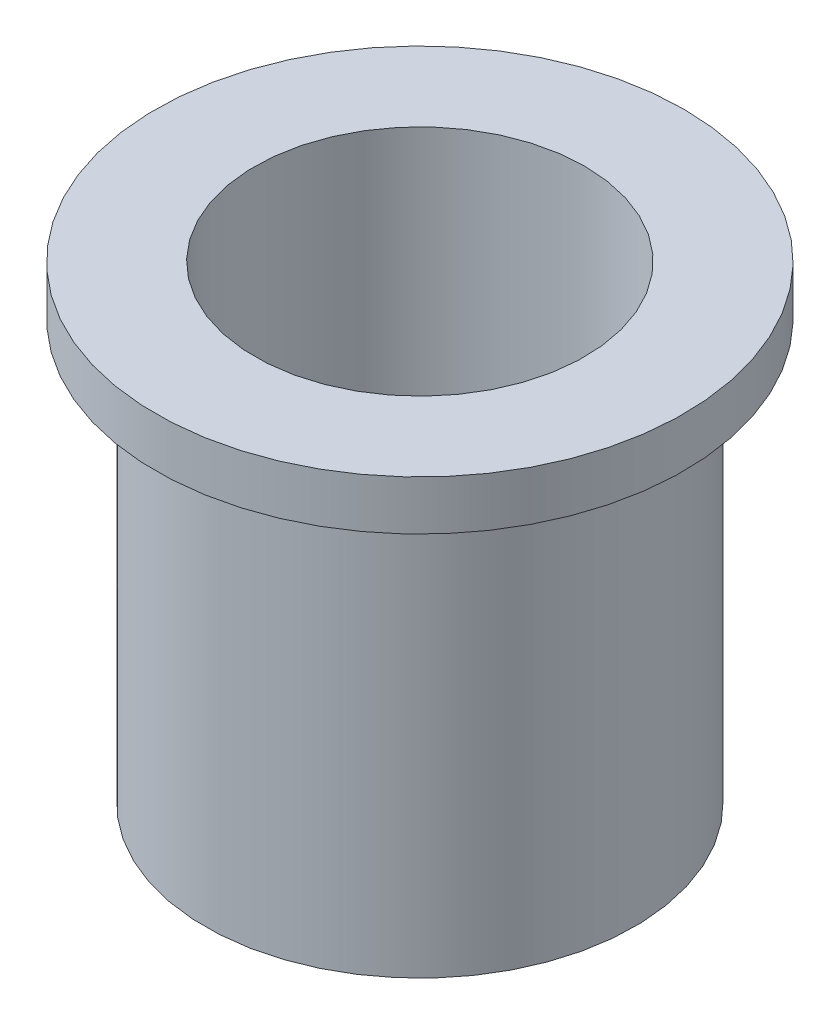
# Autodesk Inventor part: Flange_Bearing_5448T5
Saved by Autodesk Inventor 2015 (Build 190159000, 159)
## iProperties
Created: 2014-12-22
Part Number: Flange_Bearing_5448T5
Material: Generic
Document SubType Name: Modeling
Designer: Drew
Density: 1 g/cm^3
Appearance: Default
Author: Drew
Autodesk Inventor part; units mm, degrees
ref_plane "YZ Plane" through (0, 0, 0) normal (1, 0, 0) x (0, 1, 0)
ref_plane "XZ Plane" through (0, 0, 0) normal (0, 1, 0) x (-1, 0, 0)
ref_plane "XY Plane" through (0, 0, 0) normal (0, 0, 1) x (1, 0, 0)
sketch "Sketch1" plane through (0, 0, 0) normal (1, 0, 0) x (0, 1, 0)
  line L0 (0, -5) -> (-14.2162, -5)
  line L1 (-14.2162, -5) -> (-14.2162, -6.5)
  line L2 (-14.2162, -6.5) -> (-1.5, -6.5)
  line L3 (-1.5, -6.5) -> (-1.5, -8)
  line L4 (-1.5, -8) -> (0, -8)
  line L5 (0, -8) -> (0, -5)
  line L6 (6.1756, 0) -> (-16.6954, 0)
  point P0 (0, 0)
  dimension "d1" = 10
  dimension "d3" = 13
  dimension "d4" = 1.5
  dimension "d5" = 16
  constraints: 14 end point, 5 perpendicular, 2 horizontal, 1 point on line
  measures "d1" diameter of L0 L6
  measures "d3" diameter of L2 L6
  measures "d4" distance between parallel lines of L5 L3
  measures "d5" diameter of L4 L6
revolve "Revolution1" add sketch "Sketch1" angle 360 about axis through (0, 6.1756, 0) along (0, -1, 0)
body "Solid1"
